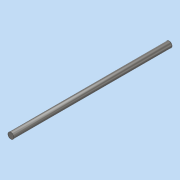
# Autodesk Inventor part: Shaft
Saved by Autodesk Inventor 2017 (Build 210142000, 142)
## iProperties
Created: 2017-04-13
Part Number: Shaft
Material: Stainless Steel
Document SubType Name: Modeling
Designer: Derek
Density: 8 g/cm^3
Appearance: Semi-Polished
Mass: 18.099 g
Surface Area: 19.3578 cm^2
Volume: 2.26237 cm^3
Author: Derek Wider
Autodesk Inventor part; units mm, degrees
ref_plane "YZ Plane" through (0, 0, 0) normal (1, 0, 0) x (0, 1, 0)
ref_plane "XZ Plane" through (0, 0, 0) normal (0, 1, 0) x (-1, 0, 0)
ref_plane "XY Plane" through (0, 0, 0) normal (0, 0, 1) x (1, 0, 0)
sketch "Sketch1" plane through (0, 0, 0) normal (0, 0, 1) x (1, 0, 0)
  circle A0 centre (0, 0) radius 2.3813
  dimension "d0" = 4.7625
  constraints: 1 centre point, 1 coincident
  measures "d0" diameter of A0
extrude "Extrusion1" add sketch "Sketch1" along normal blind 127
body "Solid1"
